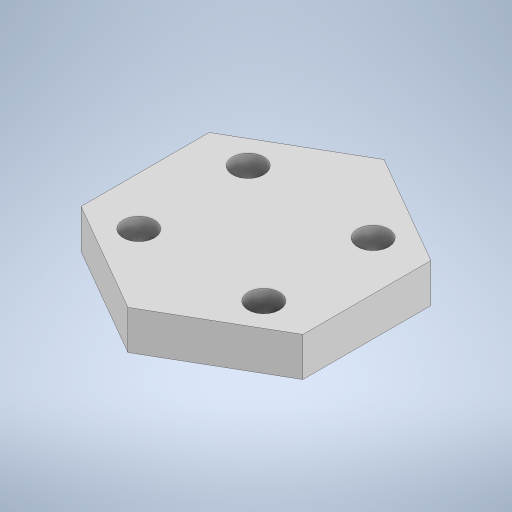
# Autodesk Inventor part: WH-SuspensionBounding-FirstApproach
Saved by Autodesk Inventor 2024.2 (Build 282272000, 272)
## iProperties
Created: 2025-07-14
Part Number: WH-SuspensionBounding-FirstApproach
Material: Generic
Document SubType Name: Modeling
Designer: Admin
Density: 1 g/cm^3
Appearance: Default
Author: Admin
Autodesk Inventor part; units mm, degrees
ref_plane "YZ Plane" through (0, 0, 0) normal (1, 0, 0) x (0, 1, 0)
ref_plane "XZ Plane" through (0, 0, 0) normal (0, 1, 0) x (-1, 0, 0)
ref_plane "XY Plane" through (0, 0, 0) normal (0, 0, 1) x (1, 0, 0)
sketch "Sketch1" plane through (0, 0, 0) normal (0, 1, 0) x (-1, 0, 0)
  circle A0 centre (8, -7) radius 2
  line L0 (8, -7) -> (8, 7) construction
  circle A1 centre (8, 7) radius 2
  line L1 (0, 0) -> (0, -15) construction
  circle A2 centre (-8, -7) radius 2
  circle A3 centre (-8, 7) radius 2
  line L2 (0, 16.3959) -> (14.1992, 8.1979)
  line L3 (14.1992, 8.1979) -> (14.1992, -8.1979)
  line L4 (14.1992, -8.1979) -> (0, -16.3959)
  line L5 (0, -16.3959) -> (-14.1992, -8.1979)
  line L6 (-14.1992, -8.1979) -> (-14.1992, 8.1979)
  line L7 (-14.1992, 8.1979) -> (0, 16.3959)
  dimension "d0" = 7
  dimension "d2" = 4
  dimension "d3" = 8
  dimension "d4" = 14
  dimension "d5" = 4
  dimension "d7" = 15
  constraints: 16 end point, 4 centre point, 3 coincident, 2 symmetric about line, 2 vertical, 1 point on line, 15 other
  measures "d0" vertical distance of L0.start point (0, 0)
  measures "d2" diameter of A0
  measures "d3" horizontal distance of point (0, 0) L0.start
  measures "d4" distance of L0.start L0.end
  measures "d5" diameter of A1
  measures "d7" distance of L1.start L1.end
extrude "Extrusion1" add sketch "Sketch1" along normal blind 5
body "Solid1"
